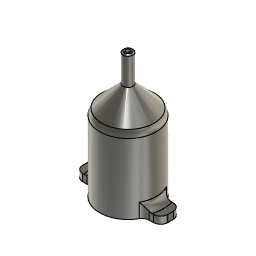
3D_prentun_hlutur_sprauta (Autodesk Fusion 360 design; units mm, degrees)
Autodesk Fusion 360 part; units mm, degrees
note: some values were not read from the file. Chosen so that the rebuilt part matches the saved one: which bodies a step acts on; which face or edge a step refers to; which pieces of a blend or face edit are solid. Set by a fixed rule: which sketch regions a step uses.
sketch "Sketch1" plane through (0, 0, 0) normal (0, 0, 1) x (1, 0, 0)
  circle A0 centre (0, 0) radius 20
  dimension "d6" = 40
  constraint coincident A0.centre origin
  measures "d6" diameter of A0
extrude "Extrude1" add sketch "Sketch1" along normal blind 50 makes body 1
sketch "Sketch2" plane through (0, 0, 0) normal (0, 0, -1) x (1, 0, 0)
  circle A0 centre (0, 0) radius 20
  circle A1 centre (0, 0) radius 16
extrude "Extrude2" cut sketch "Sketch2" against normal blind 46 contours A1 bodies 1
sketch "Sketch3" plane through (0, 0, 50) normal (0, 0, 1) x (-1, 0, 0)
  circle A0 centre (0, 0) radius 20
  circle A1 centre (0, 0) radius 3.5
  dimension "d14" = 7
  constraint concentric A0 A1
  measures "d14" diameter of A1
extrude "Extrude3" add sketch "Sketch3" along normal blind 30 contours A1 bodies 1
sketch "Sketch4" plane through (0, 0, 80) normal (0, 0, 1) x (-1, 0, 0)
  circle A0 centre (0, 0) radius 3.5
  circle A1 centre (0, 0) radius 1.5
extrude "Extrude4" cut sketch "Sketch4" against normal blind 34 contours A1 bodies 1
sketch "Sketch5" plane through (0, 0, 46) normal (0, 0, -1) x (1, 0, 0)
  circle A0 centre (0, 0) radius 16
  circle A1 centre (0, 0) radius 16
  circle A2 centre (0, 0) radius 16
  circle A3 centre (0, 0) radius 15.7
  circle A4 centre (0, 0) radius 1.5
  dimension "d20" = 31.4
  constraint concentric A2 A3
  measures "d20" diameter of A3
extrude "Extrude5" add sketch "Sketch5" along normal blind 4 separate body contours A3 | A4 makes body 2
sketch "Sketch6" plane through (0, 0, 42) normal (0, 0, -1) x (1, 0, 0)
  circle A0 centre (0, 0) radius 15.7
  circle A1 centre (0, 0) radius 3.5
  dimension "d26" = 7
  constraint concentric A0 A1
  measures "d26" diameter of A1
extrude "Extrude6" add sketch "Sketch6" along normal blind 46.6 contours A1 bodies 2
sketch "Sketch7" plane through (0, 0, -4.6) normal (0, 0, -1) x (1, 0, 0)
  circle A0 centre (0, 0) radius 3.5
  circle A1 centre (0, 0) radius 10
  dimension "d30" = 20
  constraint coincident A0.centre A1.centre
  measures "d30" diameter of A1
extrude "Extrude7" add sketch "Sketch7" along normal blind 4 contours A0 | A1 bodies 2
sketch "Sketch8" plane through (0, 0, 0) normal (0, 0, -1) x (1, 0, 0)
  circle A0 centre (0, 0) radius 16
  circle A1 centre (0, 0) radius 20
  circle A2 centre (0, 0) radius 20
  circle A3 centre (0, 0) radius 3.8
  dimension "d34" = 40
  dimension "d35" = 7.6
  constraint concentric A0 A2
  constraint concentric A2 A3
  measures "d34" diameter of A2
  measures "d35" diameter of A3
extrude "Extrude8" add sketch "Sketch8" along normal blind 4 contours A0 | A1 A2 bodies 1
sketch "Sketch9" plane through (0, 0, 0) normal (0, 1, 0) x (1, 0, 0)
  line L0 (0, 0) -> (0, -60) construction
  line L1 (15.7, -42) -> (-15.7, -42)
  line L2 (3.5, 4.6) -> (-3.5, 4.6)
  line L3 (-3.5, -42) -> (3.5, -42)
  line L4 (15.7, -42) -> (3.5, -29.8)
  line L5 (15.7, -42) -> (30.9528, -42) construction
  line L6 (3.5, -29.8) -> (3.5, -42)
  line L7 (15.7, -42) -> (3.5, -42)
  dimension "d42" = 135
  constraint coincident L0.start origin
  constraint vertical L0
  constraint horizontal L5
  constraint coincident L1.start L4.start
  constraint coincident L3.end L6.end
  constraint perpendicular L1 L6
  measures "d42" angle of L4 L5
revolve "Revolve1" add sketch "Sketch9" angle 360 about axis through (0, 0, 0) along (0, 0, 1) bodies 2
sketch "Sketch10" plane through (0, 0, 0) normal (0, 1, 0) x (1, 0, 0)
  line L0 (-3.8, 0) -> (3.8, 0)
  line L1 (-16, 0) -> (16, 0)
  line L2 (16, 0) -> (16, -12.2)
  line L3 (3.8, 0) -> (16, 0)
  line L4 (3.8, 0) -> (16, -12.2)
  dimension "d45" = 45
  constraint coincident L0.end L3.start
  constraint coincident L1.end L2.start
  constraint perpendicular L1 L2
  measures "d45" angle of L3 L4
revolve "Revolve2" add sketch "Sketch10" angle 360 about axis through (0, 0, 1.75) along (0, 0, 1) bodies 1
sketch "Sketch11" plane through (0, 0, -4) normal (0, 0, -1) x (1, 0, 0)
  circle A0 centre (0, 0) radius 3.8
  circle A1 centre (0, 0) radius 20
  line L0 (30, 7) -> (-30, 7)
  line L1 (-30, 7) -> (-30, -7)
  line L2 (-30, -7) -> (30, -7)
  line L3 (30, -7) -> (30, 7)
  line L4 (30, 7) -> (-30, -7) construction
  line L5 (-30, 7) -> (30, -7) construction
  dimension "d47" = 60
  dimension "d48" = 14
  constraint horizontal L0
  constraint perpendicular L0 L1
  constraint parallel L0 L2
  constraint parallel L1 L3
  constraint coincident L4 A0.centre
  constraint coincident L5 A0.centre
  constraint coincident A0.centre A1.centre
  measures "d47" distance of L1.end L2.end
  measures "d48" distance of L0.start L2.end
extrude "Extrude9" add sketch "Sketch11" against normal blind 5 contours A1 L0 L2 L3 | A1 L0 L1 L2 bodies 1
fillet "Fillet1" radius 5 4 edges at (30, 7, -1.5) (30, -7, -1.5) (-30, 7, -1.5) (-30, -7, -1.5) on bodies 1
fillet "Fillet2" radius 5 4 edges at (18.735, 7, -1.5) (18.735, -7, -1.5) (-18.735, -7, -1.5) (-18.735, 7, -1.5) on bodies 1
fillet "Fillet3" radius 5 2 edges at (20, 0, 1) (-20, 0, 1) on bodies 1
sketch "Sketch12" plane through (0, 0, 0) normal (0, 1, 0) x (1, 0, 0)
  line L0 (-20, -50) -> (20, -50)
  line L1 (-3.5, -80) -> (3.5, -80)
  line L2 (3.5, -50) -> (-3.5, -50)
  line L3 (3.5, -50) -> (18.5, -50)
  line L4 (18.5, -50) -> (3.5, -65)
  line L5 (3.5, -50) -> (3.5, -80)
  dimension "d68" = 45
  dimension "d70" = 15
  constraint coincident L2.start L3.start
  constraint coincident L0 L3.end
  constraint parallel L0 L3
  constraint coincident L1.end L5.end
  constraint coincident L4.end L5
  measures "d68" angle of L3 L4
  measures "d70" distance of L2.start L3.end
revolve "Revolve3" add sketch "Sketch12" angle 360 about axis through (0, 0, 1.75) along (0, 0, 1) bodies 1
chamfer "Chamfer4" distance 14.5 angle 45 1 edges at (1.3985, 0.5424, 46) on bodies 1
extrude "Extrude10" add 1 faces at (-5.0008, -1.5426, 46) along direction (0, 0, 1) blind 14.5 separate body on bodies 2 makes body 3
combine "Combine1" operation add target body 3 tool bodies 2
combine "Combine2" operation cut target body 3 tool bodies 1 keep tools makes body 4 at (-5.1107, -13.0219, 54.5111)
fillet "Fillet5" radius 7.5 1 edges at (-18.6465, -7.2323, 50) on bodies 1
extrude "Extrude11" add 1 faces at (-2.8203, 0.1739, 80) along direction (0, 0, 1) blind 5 on bodies 1 bodies 1
move_body "Move5" bodies 3 to x (1, 0, 0) y (0, 1, 0) z (0, 0, 1) at (0, 0, -0.8)
delete_body "RemoveBody1" bodies 4
chamfer "Chamfer5" distance 1 angle 45 1 edges at (3.2631, 1.2657, 85) on bodies 1
equation "adal_R = 40 mm"
equation "h = 50 mm"
equation "op_h = 30 mm"
equation "d = 7 mm"
equation "d_offset = 2 mm"
equation "d6 = adal_R"
equation "adal_R_offset = 4 mm"
equation "d8 = h"
equation "d10 = -adal_R_offset"
equation "dypt = h - adal_R_offset"
equation "d12 = -dypt"
equation "d14 = d"
equation "d15 = op_h"
equation "d17 = -d_offset"
equation "d20 = adal_R - ( TOL + 2 * adal_R_offset )"
equation "TOL = 0.6 mm"
equation "sprautu_botn_thykkt = 4 mm"
equation "d23 = sprautu_botn_thykkt"
equation "sprautu_bar_d = 7 mm"
equation "d26 = sprautu_bar_d"
equation "d27 = sprautu_bar_h"
equation "sprautu_bar_h = h + TOL - adal_R_offset"
equation "d31 = sprautu_push_thykkt"
equation "sprautu_push_thykkt = 4 mm"
equation "d34 = adal_R"
equation "d35 = sprautu_bar_d + TOL"
equation "BOTN_thykkt = 4 mm"
equation "d37 = adal_R_offset"
equation "d47 = adal_R * 1.5"
equation "d48 = 2 * sprautu_bar_d"
equation "d49 = -handlebar_thykkt"
equation "handlebar_thykkt = 5 mm"
equation "handlebarfillet = 5 mm"
equation "d54 = handlebarfillet"
equation "d56 = handlebarfillet"
equation "d58 = handlebarfillet"
equation "sprautu_toppur_fillet = 15 mm"
equation "d63 = sprautu_toppur_fillet / 2"
equation "sprautu_push_d = 20 mm"
equation "d68 = horn"
equation "horn = 45 deg"
equation "d70 = efra_sprautu_chamfer"
equation "efra_sprautu_chamfer = 15 mm"
